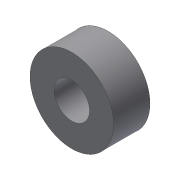
# Autodesk Inventor part: UPPER_TIMING_PULLEY_COVER_INNER
Saved by Autodesk Inventor 2019.4 (Build 234330000, 330)
## iProperties
Created: 2019-11-13
Part Number: UPPER_TIMING_PULLEY_COVER_INNER
Material: 一般
Document SubType Name: Modeling
Designer: y6tada
Density: 1 g/cm^3
Appearance: Black 100
Author: y6tada
Autodesk Inventor part; units mm, degrees
ref_plane "YZ Plane" through (0, 0, 0) normal (1, 0, 0) x (0, 1, 0)
ref_plane "XZ Plane" through (0, 0, 0) normal (0, 1, 0) x (-1, 0, 0)
ref_plane "XY Plane" through (0, 0, 0) normal (0, 0, 1) x (1, 0, 0)
sketch "スケッチ1" plane through (0, 0, 0) normal (0, 0, 1) x (1, 0, 0)
  circle A0 centre (0, 0) radius 14.05
  circle A1 centre (0, 0) radius 19.97 projected
  circle A2 centre (0, 0) radius 14 construction
  point P0 (0, 0)
  dimension "d2" = 0.05
  constraints: 1 centre point, 1 concentric
  measures "d2" radial gap between concentric circles of A2 A0
extrude "押し出し1" add sketch "スケッチ1" along normal blind 1
chamfer "面取り1" distance 0.4 angle 45 1 edges at (-19.97, 0, 0)
sketch "スケッチ2" plane through (0, 0, 1) normal (0, 0, 1) x (1, 0, 0)
  circle A0 centre (6.1229, -14.7821) radius 0.5915 construction
  point P0 (0, 0)
  point P1 (14.7821, -6.1229)
  point P2 (14.7821, 6.1229)
  point P3 (6.1229, 14.7821)
  point P4 (-6.1229, 14.7821)
  point P5 (-14.7821, 6.1229)
  point P6 (-14.7821, -6.1229)
  point P7 (-6.1229, -14.7821)
  dimension "d8" = 360
  constraints: 1 coincident, 9 other
hole "穴1" at (6.1229, -14.7821, 1) at (14.7821, -6.1229, 1) at (14.7821, 6.1229, 1) at (6.1229, 14.7821, 1) at (-6.1229, 14.7821, 1) at (-14.7821, 6.1229, 1) at (-14.7821, -6.1229, 1) at (-6.1229, -14.7821, 1) direction (0, 0, -1) diameter 1.4 end through all countersink diameter 2.2 countersink angle 82
